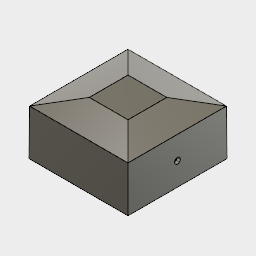
Crazyfire HZ-100P Housing v4 (Autodesk Fusion 360 design; units mm, degrees)
Autodesk Fusion 360 part; units mm, degrees
sketch "Sketch1" plane through (0, 0, 0) normal (0, 0, 1) x (1, 0, 0)
  line L0 (-21.1, 19.5) -> (21.1, 19.5) construction
  line L1 (21.1, 19.5) -> (21.25, 0)
  line L2 (21.25, 0) -> (-21.25, 0)
  line L3 (-21.25, 0) -> (-21.1, 19.5)
  line L4 (0, 0) -> (0, 61.8578) construction
  line L5 (-8.3, 22.7) -> (8.3, 22.7)
  line L6 (-8.3, 22.7) -> (-21.1, 19.5)
  line L7 (8.3, 22.7) -> (21.1, 19.5)
  point P0 (0, 22.7)
  dimension "d1" = 16.6
  dimension "d2" = 42.5
  dimension "d3" = 42.2
  dimension "d4" = 19.5
  dimension "d5" = 22.7
  measures "d1" distance of L5.start L5.end
  measures "d2" distance of L2.start L2.end L1
  measures "d3" distance of L0.start L0.end
  measures "d4" distance of L0 L2 L1
  measures "d5" distance of L2 L5 L1
extrude "Extrude1" add sketch "Sketch1" along normal blind 90 makes body 1
copy_body "CopyPasteBodies1" bodies 1 makes body 2
move_body "Move1" bodies 2 to x (0, 0, -1) y (0, 1, 0) z (1, 0, 0) at (-45, 0, 45)
combine "Combine1" operation intersect target body 2 tool bodies 1
shell "Shell1" thickness 1.4 removed faces 1 at (7.0833, 0, 37.9167) on bodies 2
ref_plane "WorkPlane1" through (0, 16.4, 45) normal (0, -1, 0) x (0, 0, -1)
sketch "Sketch3" plane through (-21.2487, 0.1635, 0) normal (-0.99997, 0.007692, 0) x (0, 0, 1)
  line L0 (23.9, 19.3371) -> (23.75, -0.1635)
  line L1 (23.75, -0.1635) -> (66.25, -0.1635)
  line L2 (66.25, -0.1635) -> (66.1, 19.3371)
  line L3 (66.1, 19.3371) -> (23.9, 19.3371)
  circle A0 centre (45, 9.5868) radius 1.25
  line L4 (45, -0.1635) -> (45, 19.3371) construction
  point P0 (45, 9.5868)
  dimension "d13" = 2.5
  measures "d13" diameter of A0
extrude "Extrude2" cut sketch "Sketch3" against normal blind 6 contours A0 bodies 2
sketch "Sketch4" plane through (21.2487, 0.1635, 0) normal (0.99997, 0.007692, 0) x (0, 0, -1)
  line L0 (-23.75, -0.1635) -> (-23.9, 19.3371)
  line L1 (-23.9, 19.3371) -> (-66.1, 19.3371)
  line L2 (-66.1, 19.3371) -> (-66.25, -0.1635)
  line L3 (-66.25, -0.1635) -> (-23.75, -0.1635)
  circle A0 centre (-45, 9.5868) radius 1.25
  line L4 (-45, -0.1635) -> (-45, 19.3371) construction
  dimension "d16" = 2.5
  measures "d16" diameter of A0
extrude "Extrude3" cut sketch "Sketch4" against normal blind 11 contours A0 bodies 2
